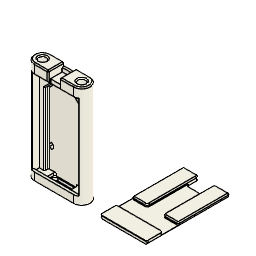
shuffle-holder (Autodesk Fusion 360 design; units mm, degrees)
Autodesk Fusion 360 part; units mm, degrees
sketch "shuffle-01" plane through (0, 0, 0) normal (0, 0, 1) x (1, 0, 0)
  line L0 (-5, 7) -> (-5, 5.4) construction
  line L1 (-7, 7.15) -> (-5, 7.15)
  line L2 (-5, 5.35) -> (-23, 5.35)
  line L3 (-21, 7.15) -> (-21, 10.2)
  line L4 (-16.25, 4.75) -> (-16.25, 9.25) construction
  line L5 (-23, 7) -> (-5, 7) construction
  line L6 (-11.75, 9.25) -> (-11.75, 4.75) construction
  line L7 (-21.6, 10.2) -> (-6.4, 10.2)
  circle A0 centre (-6.4, 7) radius 1.425
  line L8 (-7, 8.7) -> (-21, 8.7)
  line L9 (-23, 7.15) -> (-21, 7.15)
  arc A1 (-16.925, 8.3) -> (-16.925, 5.7) centre (-16.925, 7) ccw
  line L10 (-16.25, 10.2) -> (-16.25, 3.8)
  line L11 (-16.25, 9.25) -> (-11.75, 9.25) construction
  line L12 (-18.55, 5.35) -> (-18.55, 8.7)
  arc A2 (-21.6, 10.2) -> (-21.6, 3.8) centre (-21.6, 7) ccw
  arc A3 (-11.075, 5.7) -> (-11.075, 8.3) centre (-11.075, 7) ccw
  line L13 (-16.925, 8.3) -> (-11.075, 8.3)
  line L14 (-16.25, 9.3) -> (-11.75, 9.3)
  line L15 (-21.6, 3.8) -> (-6.4, 3.8)
  line L16 (-23, 5.4) -> (-5, 5.4) construction
  line L17 (-7, 7.15) -> (-7, 10.2)
  arc A4 (-6.4, 3.8) -> (-6.4, 10.2) centre (-6.4, 7) ccw
  circle A5 centre (-21.6, 7) radius 1.425
  line L18 (-9.45, 8.7) -> (-9.45, 5.35)
  circle A6 centre (-14, 7) radius 1.4 construction
  line L19 (-23, 7) -> (-23, 5.4) construction
  line L20 (-11.75, 10.2) -> (-11.75, 3.8)
  line L21 (-11.75, 4.75) -> (-16.25, 4.75) construction
  line L22 (-16.25, 4.7) -> (-11.75, 4.7)
  line L23 (-16.925, 5.7) -> (-11.075, 5.7)
  line L24 (-5, 4.1225) -> (-5, 7.15)
  line L25 (-23, 4.1225) -> (-23, 7.15)
  line L26 (16, 16.1) -> (22, 16.1)
  line L27 (4, 16.1) -> (10, 16.1)
  line L28 (10, 36.2) -> (4, 36.2)
  line L29 (16, 36.2) -> (16, 16.1)
  line L30 (4, 36.2) -> (4, 4.1)
  line L31 (10, 36.2) -> (10, 16.1)
  line L32 (22, 10.1) -> (4, 10.1)
  line L33 (10, 31.1) -> (16, 31.1)
  line L34 (4, 4.1) -> (22, 4.1)
  line L35 (22, 36.2) -> (16, 36.2)
  line L36 (22, 4.1) -> (22, 36.2)
  line L37 (4, 4.1) -> (4, 3.8)
  line L38 (4, 3.8) -> (22, 3.8)
  line L39 (22, 3.8) -> (22, 4.1)
  point P0 (-14, 7)
  point P1 (-14, 7)
  dimension "d1" = 2.8
  dimension "d2" = 2.85
  dimension "d3" = 2.85
  constraint coincident P0 A6.centre
  constraint collinear L1 L9
  constraint coincident L3.end L7
  constraint coincident L17.end L7
  constraint horizontal L21
  constraint perpendicular L4 L21
  constraint parallel L11 L21
  constraint parallel L4 L6
  constraint coincident P1 P0
  constraint coincident A2.centre A5.centre
  constraint coincident A0.centre A4.centre
  constraint coincident L10.start L7
  constraint coincident L10.end L15
  constraint perpendicular L10 L15
  constraint coincident L20.start L7
  constraint coincident L20.end L15
  constraint perpendicular L15 L20
  constraint coincident L14.start L10
  constraint coincident L14.end L20
  constraint perpendicular L14 L20
  constraint perpendicular L3 L8
  constraint coincident L8.end L3
  constraint coincident L22.start L10
  constraint coincident L22.end L20
  constraint perpendicular L20 L22
  constraint coincident L8.start L17
  constraint coincident L12.end L8
  constraint coincident L12.start L2
  constraint coincident L18.end L2
  constraint coincident L18.start L8
  constraint coincident A1.centre L5
  constraint coincident A3.centre L5
  constraint tangent A3 L23
  constraint tangent A3 L13
  constraint perpendicular L1 L24
  constraint coincident A4 L24.start
  constraint coincident L24 L2.start
  constraint perpendicular L9 L25
  constraint coincident L25 L2.end
  constraint coincident A2 L25.start
  constraint horizontal L34
  constraint vertical L36
  constraint horizontal L35
  constraint vertical L30
  constraint coincident L32.end L30
  constraint coincident L32.start L36
  constraint perpendicular L30 L32
  constraint perpendicular L29 L32
  constraint coincident L27.start L30
  constraint perpendicular L27 L31
  constraint coincident L26.start L27
  constraint collinear L26 L27
  constraint coincident L33.start L31
  constraint coincident L33.end L29
  constraint perpendicular L29 L33
  constraint collinear L28 L35
  constraint perpendicular L34 L37
  constraint perpendicular L36 L38
  constraint perpendicular L34 L39
  measures "d1" diameter of A6
  measures "d2" diameter of A5
  measures "d3" diameter of A0
extrude "Extrude1" add sketch "shuffle-01" along normal blind 1 contours L2 L8 A3 L13 L18 L20 L23 | L8 L10 L13 L20 | L2 L10 L20 L23 | L2 L8 A1 L10 L12 L13 L23 makes body 1
extrude "Extrude2" add sketch "shuffle-01" along normal blind 2 contours L1 A0 L17 L24 | L2 A0 L8 L17 L18 L24 | L2 L3 L8 L12 A5 L25 | L3 L9 A5 L25 picked at (-5.6667, 7.0114) picked at (-22.3333, 7.0114) bodies 1
extrude "Extrude3" add sketch "shuffle-01" along normal blind 3 contours L2 L15 A4 L20 L24 | L2 L10 L20 L22 | L2 L10 A2 L15 L25 | L10 L15 L20 L22 bodies 1
extrude "Extrude4" add sketch "shuffle-01" along normal blind 39.6 contours L1 A0 L17 L24 | L7 A0 L17 A4 L24 | L3 L7 A2 A5 L25 | L3 L9 A5 L25 picked at (-5.6777, 7.2342) picked at (-22.3047, 7.2838) bodies 1
extrude "Extrude5" add sketch "shuffle-01" along normal blind 4.5 from surface at 35.1 contours L1 A0 L17 L24 | L2 A0 L8 L17 L18 L24 | L7 L8 L17 L20 | L2 L15 A4 L20 L24 | L2 L8 A3 L13 L18 L20 L23 | L2 L8 A1 L10 L12 L13 L23 | L3 L7 L8 L10 | A3 L13 L20 L23 | L2 L10 A2 L15 L25 | L2 L3 L8 L12 A5 L25 | A1 L10 L13 L23 | L3 L9 A5 L25 picked at (-5.6667, 7.0114) picked at (-22.3333, 7.0114) bodies 1
extrude "Extrude11" add sketch "shuffle-01" along normal blind 3 from surface at 35.1 contours L7 L10 L14 L20 bodies 1
extrude "Extrude6" add sketch "shuffle-01" along normal blind 1.5 from surface at 35.1 contours L8 L10 L13 L20 | L8 L10 L14 L20 | L2 L10 L20 L22 | L2 L10 L20 L23 | L10 L13 L20 L23 bodies 1
extrude "Extrude7" add sketch "shuffle-01" along normal blind 35.1 contours L7 L8 L17 L20 | L8 L10 L14 L20 | L7 L10 L14 L20 | L3 L7 L8 L10 bodies 1
extrude "Extrude8" cut sketch "shuffle-01" along normal blind 3.5 from surface at 36.1 contours L1 A0 L17 L24 | L1 A0 L17 L24 | L3 L9 A5 L25 | L3 L9 A5 L25 bodies 1
sketch "shuffle-02" plane through (0, 8.7, 0) normal (0, -1, 0) x (1, 0, 0)
  line L0 (-21, 2) -> (-18.55, 2)
  line L1 (-18.55, 2) -> (-18.55, 1)
  line L2 (-18.55, 1) -> (-9.45, 1)
  line L3 (-9.45, 1) -> (-9.45, 2)
  line L4 (-9.45, 2) -> (-7, 2)
  line L5 (-7, 2) -> (-7, 35.1)
  line L6 (-7, 35.1) -> (-21, 35.1)
  line L7 (-21, 35.1) -> (-21, 2)
  line L8 (-9.5, 32.4) -> (-18.5, 32.4)
  line L9 (-18.5, 32.4) -> (-18.5, 35.1)
  line L10 (-18.5, 35.1) -> (-9.5, 35.1)
  line L11 (-9.5, 35.1) -> (-9.5, 32.4)
  line L12 (-18.5, 32.4) -> (-21, 32.4)
  line L13 (-9.5, 32.4) -> (-7, 32.4)
  line L14 (-20.5, 9) -> (-20.5, 11.4)
  line L15 (-20.5, 11.4) -> (-19.1, 11.4)
  line L16 (-19.1, 11.4) -> (-19.1, 9)
  line L17 (-19.1, 9) -> (-20.5, 9)
  line L18 (-7.5, 9) -> (-7.5, 11.4)
  line L19 (-7.5, 11.4) -> (-8.9, 11.4)
  line L20 (-8.9, 11.4) -> (-8.9, 9)
  line L21 (-8.9, 9) -> (-7.5, 9)
  point P0 (-14, 33.75)
  constraint horizontal L8
  constraint perpendicular L8 L9
  constraint parallel L8 L10
  constraint parallel L9 L11
  constraint coincident L7 L12.end
  constraint perpendicular L7 L12
  constraint coincident L5 L13.end
  constraint perpendicular L5 L13
  constraint perpendicular L7 L15
  constraint perpendicular L14 L17
  constraint perpendicular L17 L18
  constraint perpendicular L5 L19
  constraint perpendicular L18 L21
extrude "Extrude9" cut sketch "shuffle-02" against normal blind 1.5 contours L6 L8 L9 L10 L11 | L14 L15 L16 L17 | L18 L19 L20 L21 bodies 1
extrude "Extrude10" add sketch "shuffle-02" along normal blind 1.55 contours L6 L7 L9 L12 | L5 L6 L11 L13 bodies 1
chamfer "Chamfer1" distance 2.5 angle 45 2 edges at (-21, 7.925, 32.4) (-7, 7.925, 32.4) on bodies 1
fillet "Fillet1" radius 0.6 4 edges at (-18.55, 8.7, 1.5) (-9.45, 8.7, 1.5) (-9.45, 5.35, 1.5) (-18.55, 5.35, 1.5) on bodies 1
chamfer "Chamfer2" distance 0.5 angle 45 1 edges at (-14, 5.35, 3) on bodies 1
chamfer "Chamfer3" distance 0.7 angle 45 8 edges at (-20.5, 9.45, 11.4) (-8.9, 9.45, 11.4) (-19.1, 9.45, 11.4) (-7.5, 9.45, 11.4) (-20.5, 9.45, 9) (-19.1, 9.45, 9) (-7.5, 9.45, 9) (-8.9, 9.45, 9) on bodies 1
chamfer "Chamfer4" distance 0.9 angle 45 4 edges at (-18.925, 3.8, 35.1) (-22.3183, 3.8817, 35.1) (-9.075, 3.8, 35.1) (-5.6817, 3.8817, 35.1) on bodies 1
fillet "Fillet9" radius 0.2 2 edges at (-16.25, 9.3, 37.35) (-11.75, 9.3, 37.35) on bodies 1
chamfer "Chamfer5" distance 0.4 angle 45 2 edges at (-22.9286, 7.5153, 39.6) (-7.7286, 7.5153, 39.6) on bodies 1
fillet "Fillet10" radius 0.4 4 edges at (-16.25, 3.8, 37.8) (-11.75, 3.8, 37.8) (-16.25, 10.2, 38.85) (-11.75, 10.2, 38.85) on bodies 1
chamfer "Chamfer7" distance 0.4 angle 45 12 edges at (-19.125, 3.8, 39.6) (-16.3672, 3.9172, 39.6) (-16.25, 7, 39.6) (-16.3672, 10.0828, 39.6) (-19.125, 10.2, 39.6) (-24.8, 7, 39.6) (-8.875, 3.8, 39.6) (-3.2, 7, 39.6) (-8.875, 10.2, 39.6) (-11.6328, 10.0828, 39.6) (-11.75, 7, 39.6) (-11.6328, 3.9172, 39.6) on bodies 1
fillet "Fillet5" radius 0.4 6 edges at (-7, 7.15, 15.95) (-8.25, 7.15, 31.15) (-9.5, 7.15, 33.75) (-21, 7.15, 15.95) (-19.75, 7.15, 31.15) (-18.5, 7.15, 33.75) on bodies 1
fillet "Fillet6" radius 0.5 4 edges at (-21, 8.7, 15.95) (-19.75, 8.7, 31.15) (-8.25, 8.7, 31.15) (-7, 8.7, 15.95) on bodies 1
fillet "Fillet7" radius 0.2 2 edges at (-5, 4.1225, 19.5) (-23, 4.1225, 19.5) on bodies 1
fillet "Fillet8" radius 0.4 2 edges at (-18.5, 10.2, 33.75) (-9.5, 10.2, 33.75) on bodies 1
fillet "Fillet11" radius 0.2 2 edges at (-11.75, 4.7, 35.85) (-16.25, 4.7, 35.85) on bodies 1
extrude "Extrude12" add sketch "shuffle-01" along normal blind 1.5 separate body contours L26 L29 L35 L36 | L30 L32 L34 L36 | L27 L28 L30 L31 makes body 2 at (6, 29.5, 0) makes body 3 at (20, 22.8, 0) makes body 4 at (10, 8.1, 0)
extrude "Extrude13" add sketch "shuffle-01" along normal blind 0.6 contours L26 L27 L29 L30 L31 L32 L33 L36 bodies 2 3 4
extrude "Extrude14" add sketch "shuffle-01" along normal blind 0.5 from surface at 1 contours L34 L37 L38 L39 bodies 2
chamfer "Chamfer11" distance 0.3 angle 45 1 edges at (13, 3.8, 1) measured on face at (10, 3.8, 1.1667) on bodies 2
chamfer "Chamfer12" distance 0.5 angle 45 2 edges at (22, 20.15, 0) (4, 20.15, 0) measured on face at (22, 29.5, 0.7) measured on face at (4, 29.5, 0.7) on bodies 2
fillet "Fillet12" radius 0.6 4 edges at (22, 3.8, 1.4) (4, 3.8, 1.4) (22, 36.2, 1) (4, 36.2, 1) on bodies 2
fillet "Fillet13" radius 1 6 edges at (10, 16.1, 1.05) (16, 16.1, 1.05) (16, 36.2, 0.75) (10, 36.2, 0.75) (10, 31.1, 0.3) (16, 31.1, 0.3) on bodies 2
fillet "Fillet14" radius 0.6 4 edges at (22, 16.1, 1.05) (22, 10.1, 1.05) (4, 10.1, 1.05) (4, 16.1, 1.05) on bodies 2
chamfer "Chamfer13" distance 0.4 angle 45 8 edges at (16, 26.15, 1.5) (16.2929, 16.3929, 1.5) (19.2, 16.1, 1.5) (21.8243, 16.2757, 1.5) (22, 26.15, 1.5) (21.8243, 36.0243, 1.5) (19.2, 36.2, 1.5) (16.2929, 35.9071, 1.5) measured on face at (20, 29.1667, 1.5) measured on face at (16.9049, 16.1045, 0.9) measured on face at (20, 29.1667, 1.5) measured on face at (21.8342, 16.286, 0.9) measured on face at (20, 29.1667, 1.5) measured on face at (21.4397, 36.1987, 1) measured on face at (20, 29.1667, 1.5) measured on face at (16.3099, 35.9237, 0.5) on bodies 2
chamfer "Chamfer14" distance 0.4 angle 45 8 edges at (10, 26.15, 1.5) (9.7071, 35.9071, 1.5) (6.8, 36.2, 1.5) (4.1757, 36.0243, 1.5) (4, 26.15, 1.5) (4.1757, 16.2757, 1.5) (6.8, 16.1, 1.5) (9.7071, 16.3929, 1.5) measured on face at (6, 29.1667, 1.5) measured on face at (9.5801, 36.0146, 0.5) measured on face at (6, 29.1667, 1.5) measured on face at (4.5603, 36.1987, 1) measured on face at (6, 29.1667, 1.5) measured on face at (4.186, 16.2658, 0.9) measured on face at (6, 29.1667, 1.5) measured on face at (9.9955, 17.0049, 0.9) on bodies 2
